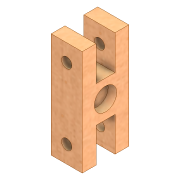
# Autodesk Inventor part: hinge
Saved by Autodesk Inventor 2020 (Build 240168000, 168)
## iProperties
Created: 2021-06-24
Part Number: hinge
Material: Generic
Document SubType Name: Modeling
Designer: Aidan Lee
Density: 1 g/cm^3
Appearance: Cherry - Natural Low Gloss
Author: Aidan Lee
Autodesk Inventor part; units mm, degrees
ref_plane "YZ Plane" through (0, 0, 0) normal (1, 0, 0) x (0, 1, 0)
ref_plane "XZ Plane" through (0, 0, 0) normal (0, 1, 0) x (-1, 0, 0)
ref_plane "XY Plane" through (0, 0, 0) normal (0, 0, 1) x (1, 0, 0)
sketch "Sketch1" plane through (0, 0, 0) normal (0, 0, 1) x (1, 0, 0)
  line L0 (0, 0) -> (18, 0)
  line L1 (18, 0) -> (18, 61)
  line L2 (18, 61) -> (0, 61)
  line L3 (0, 61) -> (0, 0)
  dimension "d0" = 18
  dimension "d1" = 61
  constraints: 8 end point, 2 parallel, 1 horizontal, 1 perpendicular
  measures "d0" distance of L1.end L2.end
  measures "d1" distance of L2.end L0.start
extrude "Extrusion1" add sketch "Sketch1" along normal blind 27
sketch "Sketch2" plane through (0, 0, 0) normal (-1, 0, 0) x (0, 0, 1)
  line L0 (0, 61) -> (27, 61) projected
  line L1 (8, 61) -> (19, 61)
  line L2 (19, 61) -> (19, 41)
  line L3 (19, 41) -> (8, 41)
  line L4 (8, 41) -> (8, 61)
  line L5 (-7.2771, 30.5) -> (-16.8885, 30.5) construction
  line L6 (0, 61) -> (0, 0) construction
  line L7 (8, 0) -> (19, 0)
  line L8 (19, 0) -> (19, 20)
  line L9 (19, 20) -> (8, 20)
  line L10 (8, 20) -> (8, 0)
  point P0 (-12.0828, 30.5)
  point P1 (0, 30.5)
  point P2 (13.5, 61)
  point P3 (13.5, 61)
  dimension "d4" = 11
  dimension "d5" = 20
  constraints: 18 end point, 4 midpoint, 4 symmetric about line, 2 horizontal, 2 parallel, 1 coincident, 1 horizontal alignment, 1 perpendicular, 1 point on line
  measures "d4" distance between parallel lines of L2 L4
  measures "d5" distance of L3.end L1.start
extrude "Extrusion2" cut sketch "Sketch2" against normal through all
sketch "Sketch3" plane through (0, 0, 27) normal (0, 0, 1) x (1, 0, 0)
  circle A0 centre (9, 51) radius 3
  line L0 (-26.5753, 30.5) -> (-43.832, 30.5) construction
  line L1 (0, 61) -> (0, 0) construction
  circle A1 centre (9, 10) radius 3
  line L2 (18, 61) -> (0, 61) construction
  line L3 (0, 41) -> (18, 41) construction
  line L4 (18, 61) -> (0, 61) construction
  line L5 (0, 61) -> (0, 41) construction
  line L6 (0, 41) -> (18, 41) construction
  line L7 (18, 41) -> (18, 61) construction
  point P0 (-35.2037, 30.5)
  point P1 (0, 30.5)
  point P2 (0, 51)
  point P3 (9, 61)
  dimension "d8" = 6
  constraints: 10 end point, 4 midpoint, 2 centre point, 2 horizontal, 2 horizontal alignment, 2 parallel, 1 perpendicular, 1 symmetric about line, 1 vertical alignment, 1 other
  measures "d8" diameter of A0
extrude "Extrusion3" cut sketch "Sketch3" against normal through all
sketch "Sketch4" plane through (18, 0, 0) normal (1, 0, 0) x (0, 0, -1)
  circle A0 centre (-13.5, 30.5) radius 6.5
  line L0 (-27, 0) -> (-27, 61) projected
  line L1 (-8, 41) -> (-19, 41) projected
  point P0 (0, 0)
  point P1 (-27, 30.5)
  point P2 (-13.5, 41)
  dimension "bearingdiameter" = 13
  constraints: 2 midpoint, 1 centre point, 1 horizontal alignment, 1 vertical alignment
  measures "bearingdiameter" diameter of A0
extrude "Extrusion4" cut sketch "Sketch4" against normal blind 5
body "Solid1"
